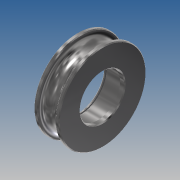
# Autodesk Inventor part: DD_KVD_004_02
Saved by Autodesk Inventor 2017.3 (Build 213256000, 256)
## iProperties
Created: 2012-08-17
Part Number: DD_KVD_004_02
Material: Nerezová ocel
Document SubType Name: Modeling
Designer: DAŘENA M.
Manufacturer: Standard
Standards Organization: Custom
Mass: 243.623 g
Surface Area: 187.558 cm^2
Volume: 30.4529 cm^3
Density: 8 g/cm^3
Appearance: Pololeštěná
HRUBA_HMOTNOST: 1,18 kg
POLOTOVAR_NORMA: ČSN 425510
ROZMER_POLOTOVARU: KR 80 - 30
Title: KLADKA ø 55
Author: DAŘENA M.
Autodesk Inventor part; units mm, degrees
ref_plane "YZ Plane" through (0, 0, 0) normal (1, 0, 0) x (0, 1, 0)
ref_plane "XZ Plane" through (0, 0, 0) normal (0, 1, 0) x (-1, 0, 0)
ref_plane "XY Plane" through (0, 0, 0) normal (0, 0, 1) x (1, 0, 0)
sketch "Náčrt1" plane through (0, 0, 0) normal (0, 0, 1) x (1, 0, 0)
  line L0 (-8, 0) -> (8, 0)
  line L1 (8, 0) -> (8, 27.5)
  line L2 (8, 27.5) -> (5.5, 27.5)
  line L3 (5.5, 27.5) -> (5.5, 26.5)
  line L4 (0.5, 21.5) -> (-0.5, 21.5)
  line L5 (-5.5, 26.5) -> (-5.5, 27.5)
  line L6 (-5.5, 27.5) -> (-8, 27.5)
  line L7 (-8, 27.5) -> (-8, 0)
  line L8 (-8, 16) -> (-6.3, 16)
  line L9 (-6.3, 16) -> (-6.3, 16.85)
  line L10 (-6.3, 16.85) -> (-5, 16.85)
  line L11 (-5, 16.85) -> (-5, 16)
  line L12 (-5, 16) -> (5, 16)
  line L13 (5, 16) -> (5, 14)
  line L14 (5, 14) -> (8, 14)
  arc A0 (-5.5, 26.5) -> (-0.5, 21.5) centre (-0.5, 26.5) ccw
  arc A1 (0.5, 21.5) -> (5.5, 26.5) centre (0.5, 26.5) ccw
  point P0 (0, 0)
  point P1 (0, 0)
  point P2 (5.5, 21.5)
  point P3 (-5.5, 21.5)
  dimension "d0" = 55
  dimension "d1" = 16
  dimension "d3" = 2.5
  dimension "d4" = 6
  dimension "d5" = 32
  dimension "d6" = 28
  dimension "d7" = 10
  dimension "d8" = 13
  dimension "d9" = 33.7
  dimension "d10" = 1.3
  dimension "d18" = 11
  dimension "d24" = 43
  dimension "d27" = 5
  constraints: 30 end point, 8 horizontal, 7 vertical, 6 point on line, 4 point on circle, 4 tangent, 3 collinear, 2 centre point, 2 coincident, 1 equal radius, 1 midpoint
  measures "d0" diameter of L1.end L0
  measures "d1" distance between parallel lines of L1 L7
  measures "d3" distance of L5.end L6.end
  measures "d4" distance of point (-5.5, 21.5) L5.end
  measures "d5" diameter of L12 L0
  measures "d6" diameter of L14 L0
  measures "d7" distance of L11.end L12.end
  measures "d8" distance from line of L7 L13.end
  measures "d9" diameter of L10 L0
  measures "d10" distance of L9.end L10.end
  measures "d18" distance of point (5.5, 21.5) point (-5.5, 21.5)
  measures "d24" diameter of L4 L0
  measures "d27" radius of A0
revolve "Rotace1" add sketch "Náčrt1" angle 360 about axis through (-8, 0, 0) along (1, 0, 0) contours L7 L6 L5 A0 L4 A1 L3 L2 L1 L14 L13 L12 L11 L10 L9 L8
chamfer "Zkosení1" distance 1 angle 45 1 edges at (-8, -16, 0)
chamfer "Zkosení2" distance 0.5 angle 45 5 edges at (-8, -27.5, 0) (-5.5, -27.5, 0) (5.5, -27.5, 0) (8, -27.5, 0) (8, -14, 0)
sketch "Náčrt2" plane through (8, 0, 0) normal (1, 0, 0) x (0, 0, -1)
  circle A0 centre (0, 0) radius 27.5 projected
  circle A1 centre (0, 0) radius 14.5 projected
  circle A2 centre (0, 0) radius 30
  dimension "d25" = 2.5
  dimension "d26" = 60
  constraints: 1 centre point, 1 coincident
  measures "d25" radial gap between concentric circles of A2 A0
  measures "d26" diameter of A2
extrude "POLOTOVAR" [suppressed]
